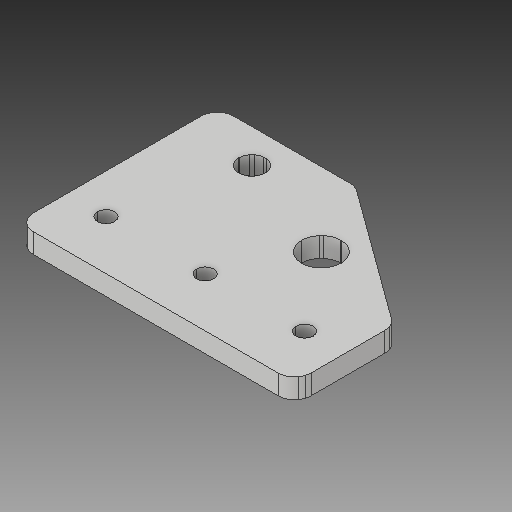
# Autodesk Inventor part: RearZHolder
Saved by Autodesk Inventor 2018 (Build 220112000, 112)
## iProperties
Created: 2016-07-23
Part Number: RearZHolder
Material: Generic
Document SubType Name: Modeling
Designer: joshm_000
Density: 1 g/cm^3
Appearance: Default
Author: joshm_000
Autodesk Inventor part; units mm, degrees
ref_plane "YZ Plane" through (0, 0, 0) normal (1, 0, 0) x (0, 1, 0)
ref_plane "XZ Plane" through (0, 0, 0) normal (0, 1, 0) x (-1, 0, 0)
ref_plane "XY Plane" through (0, 0, 0) normal (0, 0, 1) x (1, 0, 0)
sketch "Sketch1" plane through (0, 0, 0) normal (0, 1, 0) x (-1, 0, 0)
  line L0 (84.9035, 235.5734) -> (84.9035, 213.1177)
  spline S0 degree 3 poles (84.9035, 213.1177) (84.9035, 212.592) (84.9859, 212.0727) (85.1485, 211.5726) knots 1 1 1 1 2 2 2 2
  line L1 (84.9035, 213.1177) -> (84.9035, 212.592) construction
  line L2 (84.9035, 212.592) -> (84.9859, 212.0727) construction
  line L3 (84.9859, 212.0727) -> (85.1485, 211.5726) construction
  spline S1 degree 3 poles (85.1485, 211.5726) (85.3107, 211.0726) (85.5495, 210.6042) (85.8585, 210.1787) knots 2 2 2 2 3 3 3 3
  line L4 (85.1485, 211.5726) -> (85.3107, 211.0726) construction
  line L5 (85.3107, 211.0726) -> (85.5495, 210.6042) construction
  line L6 (85.5495, 210.6042) -> (85.8585, 210.1787) construction
  spline S2 degree 3 poles (85.8585, 210.1787) (86.1665, 209.755) (86.5368, 209.3843) (86.9604, 209.0756) knots 3 3 3 3 4 4 4 4
  line L7 (85.8585, 210.1787) -> (86.1665, 209.755) construction
  line L8 (86.1665, 209.755) -> (86.5368, 209.3843) construction
  line L9 (86.5368, 209.3843) -> (86.9604, 209.0756) construction
  line L10 (86.9604, 209.0756) -> (125.9367, 180.6949)
  spline S3 degree 3 poles (125.9367, 180.6949) (126.3618, 180.3855) (126.83, 180.1463) (127.3299, 179.9832) knots 5 5 5 5 6 6 6 6
  line L11 (125.9367, 180.6949) -> (126.3618, 180.3855) construction
  line L12 (126.3618, 180.3855) -> (126.83, 180.1463) construction
  line L13 (126.83, 180.1463) -> (127.3299, 179.9832) construction
  spline S4 degree 3 poles (127.3299, 179.9832) (127.8315, 179.8197) (128.3524, 179.7368) (128.88, 179.7368) knots 6 6 6 6 7 7 7 7
  line L14 (127.3299, 179.9832) -> (127.8315, 179.8197) construction
  line L15 (127.8315, 179.8197) -> (128.3524, 179.7368) construction
  line L16 (128.3524, 179.7368) -> (128.88, 179.7368) construction
  line L17 (128.88, 179.7368) -> (159.2657, 179.7368)
  line L18 (159.2657, 179.7368) -> (164.1855, 179.7368)
  spline S5 degree 3 poles (164.1855, 179.7368) (164.7112, 179.7368) (165.2304, 179.8192) (165.7305, 179.9816) (166.2305, 180.144) (166.6989, 180.3828) (167.1243, 180.6918) knots 9 9 9 9 10 10 10 11 11 11 11
  line L19 (164.1855, 179.7368) -> (164.7112, 179.7368) construction
  line L20 (164.7112, 179.7368) -> (165.2304, 179.8192) construction
  line L21 (165.2304, 179.8192) -> (165.7305, 179.9816) construction
  line L22 (165.7305, 179.9816) -> (166.2305, 180.144) construction
  line L23 (166.2305, 180.144) -> (166.6989, 180.3828) construction
  line L24 (166.6989, 180.3828) -> (167.1243, 180.6918) construction
  spline S6 degree 3 poles (167.1243, 180.6918) (167.5496, 181.0008) (167.9215, 181.3726) (168.2306, 181.798) knots 11 11 11 11 12 12 12 12
  line L25 (167.1243, 180.6918) -> (167.5496, 181.0008) construction
  line L26 (167.5496, 181.0008) -> (167.9215, 181.3726) construction
  line L27 (167.9215, 181.3726) -> (168.2306, 181.798) construction
  spline S7 degree 3 poles (168.2306, 181.798) (168.5396, 182.2232) (168.7783, 182.6917) (168.9408, 183.1919) knots 12 12 12 12 13 13 13 13
  line L28 (168.2306, 181.798) -> (168.5396, 182.2232) construction
  line L29 (168.5396, 182.2232) -> (168.7783, 182.6917) construction
  line L30 (168.7783, 182.6917) -> (168.9408, 183.1919) construction
  spline S8 degree 3 poles (168.9408, 183.1919) (169.103, 183.6918) (169.1854, 184.211) (169.1854, 184.7369) knots 13 13 13 13 14 14 14 14
  line L31 (168.9408, 183.1919) -> (169.103, 183.6918) construction
  line L32 (169.103, 183.6918) -> (169.1854, 184.211) construction
  line L33 (169.1854, 184.211) -> (169.1854, 184.7369) construction
  line L34 (169.1854, 184.7369) -> (169.1854, 235.5734)
  spline S9 degree 3 poles (169.1854, 235.5734) (169.1854, 236.0991) (169.103, 236.6185) (168.9408, 237.1183) knots 15 15 15 15 16 16 16 16
  line L35 (169.1854, 235.5734) -> (169.1854, 236.0991) construction
  line L36 (169.1854, 236.0991) -> (169.103, 236.6185) construction
  line L37 (169.103, 236.6185) -> (168.9408, 237.1183) construction
  spline S10 degree 3 poles (168.9408, 237.1183) (168.7783, 237.6186) (168.5396, 238.0869) (168.2306, 238.5122) knots 16 16 16 16 17 17 17 17
  line L38 (168.9408, 237.1183) -> (168.7783, 237.6186) construction
  line L39 (168.7783, 237.6186) -> (168.5396, 238.0869) construction
  line L40 (168.5396, 238.0869) -> (168.2306, 238.5122) construction
  spline S11 degree 3 poles (168.2306, 238.5122) (167.9215, 238.9377) (167.5496, 239.3094) (167.1243, 239.6184) knots 17 17 17 17 18 18 18 18
  line L41 (168.2306, 238.5122) -> (167.9215, 238.9377) construction
  line L42 (167.9215, 238.9377) -> (167.5496, 239.3094) construction
  line L43 (167.5496, 239.3094) -> (167.1243, 239.6184) construction
  spline S12 degree 3 poles (167.1243, 239.6184) (166.6989, 239.9275) (166.2305, 240.1662) (165.7305, 240.3287) (165.2304, 240.4911) (164.7112, 240.5734) (164.1855, 240.5734) knots 18 18 18 18 19 19 19 20 20 20 20
  line L44 (167.1243, 239.6184) -> (166.6989, 239.9275) construction
  line L45 (166.6989, 239.9275) -> (166.2305, 240.1662) construction
  line L46 (166.2305, 240.1662) -> (165.7305, 240.3287) construction
  line L47 (165.7305, 240.3287) -> (165.2304, 240.4911) construction
  line L48 (165.2304, 240.4911) -> (164.7112, 240.5734) construction
  line L49 (164.7112, 240.5734) -> (164.1855, 240.5734) construction
  line L50 (164.1855, 240.5734) -> (160.1854, 240.5734)
  line L51 (160.1854, 240.5734) -> (121.7853, 240.5734)
  line L52 (121.7853, 240.5734) -> (116.8657, 240.5734)
  line L53 (116.8657, 240.5734) -> (89.9037, 240.5734)
  spline S13 degree 3 poles (89.9037, 240.5734) (89.378, 240.5734) (88.8587, 240.4911) (88.3586, 240.3287) (87.8585, 240.1662) (87.3902, 239.9275) (86.9647, 239.6184) (86.5392, 239.3094) (86.1675, 238.9377) (85.8585, 238.5122) knots 24 24 24 24 25 25 25 26 26 26 27 27 27 27
  line L54 (89.9037, 240.5734) -> (89.378, 240.5734) construction
  line L55 (89.378, 240.5734) -> (88.8587, 240.4911) construction
  line L56 (88.8587, 240.4911) -> (88.3586, 240.3287) construction
  line L57 (88.3586, 240.3287) -> (87.8585, 240.1662) construction
  line L58 (87.8585, 240.1662) -> (87.3902, 239.9275) construction
  line L59 (87.3902, 239.9275) -> (86.9647, 239.6184) construction
  line L60 (86.9647, 239.6184) -> (86.5392, 239.3094) construction
  line L61 (86.5392, 239.3094) -> (86.1675, 238.9377) construction
  line L62 (86.1675, 238.9377) -> (85.8585, 238.5122) construction
  spline S14 degree 3 poles (85.8585, 238.5122) (85.5495, 238.0869) (85.3107, 237.6186) (85.1485, 237.1183) knots 27 27 27 27 28 28 28 28
  line L63 (85.8585, 238.5122) -> (85.5495, 238.0869) construction
  line L64 (85.5495, 238.0869) -> (85.3107, 237.6186) construction
  line L65 (85.3107, 237.6186) -> (85.1485, 237.1183) construction
  spline S15 degree 3 poles (85.1485, 237.1183) (84.9859, 236.6185) (84.9035, 236.0991) (84.9035, 235.5734) knots 28 28 28 28 29 29 29 29
  line L66 (85.1485, 237.1183) -> (84.9859, 236.6185) construction
  line L67 (84.9859, 236.6185) -> (84.9035, 236.0991) construction
  line L68 (84.9035, 236.0991) -> (84.9035, 235.5734) construction
  spline S16 degree 3 poles (148.4965, 185.9511) (146.2875, 185.9511) (144.4966, 187.7419) (144.4966, 189.9512) (144.4966, 192.1602) (146.2875, 193.951) (148.4965, 193.951) (150.7057, 193.951) (152.4966, 192.1602) (152.4966, 189.9512) (152.4966, 187.7419) (150.7057, 185.9511) (148.4965, 185.9511) knots 0 0 0 0 1 1 1 2 2 2 3 3 3 4 4 4 4
  line L69 (148.4965, 185.9511) -> (146.2875, 185.9511) construction
  line L70 (146.2875, 185.9511) -> (144.4966, 187.7419) construction
  line L71 (144.4966, 187.7419) -> (144.4966, 189.9512) construction
  line L72 (144.4966, 189.9512) -> (144.4966, 192.1602) construction
  line L73 (144.4966, 192.1602) -> (146.2875, 193.951) construction
  line L74 (146.2875, 193.951) -> (148.4965, 193.951) construction
  line L75 (148.4965, 193.951) -> (150.7057, 193.951) construction
  line L76 (150.7057, 193.951) -> (152.4966, 192.1602) construction
  line L77 (152.4966, 192.1602) -> (152.4966, 189.9512) construction
  line L78 (152.4966, 189.9512) -> (152.4966, 187.7419) construction
  line L79 (152.4966, 187.7419) -> (150.7057, 185.9511) construction
  line L80 (150.7057, 185.9511) -> (148.4965, 185.9511) construction
  spline S17 degree 3 poles (96.9036, 222.9735) (95.4677, 222.9735) (94.3038, 224.1376) (94.3038, 225.5735) (94.3038, 227.0094) (95.4677, 228.1735) (96.9036, 228.1735) (98.3397, 228.1735) (99.5037, 227.0094) (99.5037, 225.5735) (99.5037, 224.1376) (98.3397, 222.9735) (96.9036, 222.9735) knots 0 0 0 0 1 1 1 2 2 2 3 3 3 4 4 4 4
  line L81 (96.9036, 222.9735) -> (95.4677, 222.9735) construction
  line L82 (95.4677, 222.9735) -> (94.3038, 224.1376) construction
  line L83 (94.3038, 224.1376) -> (94.3038, 225.5735) construction
  line L84 (94.3038, 225.5735) -> (94.3038, 227.0094) construction
  line L85 (94.3038, 227.0094) -> (95.4677, 228.1735) construction
  line L86 (95.4677, 228.1735) -> (96.9036, 228.1735) construction
  line L87 (96.9036, 228.1735) -> (98.3397, 228.1735) construction
  line L88 (98.3397, 228.1735) -> (99.5037, 227.0094) construction
  line L89 (99.5037, 227.0094) -> (99.5037, 225.5735) construction
  line L90 (99.5037, 225.5735) -> (99.5037, 224.1376) construction
  line L91 (99.5037, 224.1376) -> (98.3397, 222.9735) construction
  line L92 (98.3397, 222.9735) -> (96.9036, 222.9735) construction
  spline S18 degree 3 poles (157.1854, 222.9735) (155.7495, 222.9735) (154.5854, 224.1376) (154.5854, 225.5735) (154.5854, 227.0094) (155.7495, 228.1735) (157.1854, 228.1735) (158.6213, 228.1735) (159.7854, 227.0094) (159.7854, 225.5735) (159.7854, 224.1376) (158.6213, 222.9735) (157.1854, 222.9735) knots 0 0 0 0 1 1 1 2 2 2 3 3 3 4 4 4 4
  line L93 (157.1854, 222.9735) -> (155.7495, 222.9735) construction
  line L94 (155.7495, 222.9735) -> (154.5854, 224.1376) construction
  line L95 (154.5854, 224.1376) -> (154.5854, 225.5735) construction
  line L96 (154.5854, 225.5735) -> (154.5854, 227.0094) construction
  line L97 (154.5854, 227.0094) -> (155.7495, 228.1735) construction
  line L98 (155.7495, 228.1735) -> (157.1854, 228.1735) construction
  line L99 (157.1854, 228.1735) -> (158.6213, 228.1735) construction
  line L100 (158.6213, 228.1735) -> (159.7854, 227.0094) construction
  line L101 (159.7854, 227.0094) -> (159.7854, 225.5735) construction
  line L102 (159.7854, 225.5735) -> (159.7854, 224.1376) construction
  line L103 (159.7854, 224.1376) -> (158.6213, 222.9735) construction
  line L104 (158.6213, 222.9735) -> (157.1854, 222.9735) construction
  spline S19 degree 3 poles (127.0446, 222.9735) (125.6087, 222.9735) (124.4446, 224.1376) (124.4446, 225.5735) (124.4446, 227.0094) (125.6087, 228.1735) (127.0446, 228.1735) (128.4805, 228.1735) (129.6446, 227.0094) (129.6446, 225.5735) (129.6446, 224.1376) (128.4805, 222.9735) (127.0446, 222.9735) knots 0 0 0 0 1 1 1 2 2 2 3 3 3 4 4 4 4
  line L105 (127.0446, 222.9735) -> (125.6087, 222.9735) construction
  line L106 (125.6087, 222.9735) -> (124.4446, 224.1376) construction
  line L107 (124.4446, 224.1376) -> (124.4446, 225.5735) construction
  line L108 (124.4446, 225.5735) -> (124.4446, 227.0094) construction
  line L109 (124.4446, 227.0094) -> (125.6087, 228.1735) construction
  line L110 (125.6087, 228.1735) -> (127.0446, 228.1735) construction
  line L111 (127.0446, 228.1735) -> (128.4805, 228.1735) construction
  line L112 (128.4805, 228.1735) -> (129.6446, 227.0094) construction
  line L113 (129.6446, 227.0094) -> (129.6446, 225.5735) construction
  line L114 (129.6446, 225.5735) -> (129.6446, 224.1376) construction
  line L115 (129.6446, 224.1376) -> (128.4805, 222.9735) construction
  line L116 (128.4805, 222.9735) -> (127.0446, 222.9735) construction
  spline S20 degree 3 poles (148.4965, 186.201) (146.4255, 186.201) (144.7465, 187.88) (144.7465, 189.9512) (144.7465, 192.022) (146.4255, 193.701) (148.4965, 193.701) (150.5677, 193.701) (152.2465, 192.022) (152.2465, 189.9512) (152.2465, 187.88) (150.5677, 186.201) (148.4965, 186.201) knots 0 0 0 0 1 1 1 2 2 2 3 3 3 4 4 4 4
  line L117 (148.4965, 186.201) -> (146.4255, 186.201) construction
  line L118 (146.4255, 186.201) -> (144.7465, 187.88) construction
  line L119 (144.7465, 187.88) -> (144.7465, 189.9512) construction
  line L120 (144.7465, 189.9512) -> (144.7465, 192.022) construction
  line L121 (144.7465, 192.022) -> (146.4255, 193.701) construction
  line L122 (146.4255, 193.701) -> (148.4965, 193.701) construction
  line L123 (148.4965, 193.701) -> (150.5677, 193.701) construction
  line L124 (150.5677, 193.701) -> (152.2465, 192.022) construction
  line L125 (152.2465, 192.022) -> (152.2465, 189.9512) construction
  line L126 (152.2465, 189.9512) -> (152.2465, 187.88) construction
  line L127 (152.2465, 187.88) -> (150.5677, 186.201) construction
  line L128 (150.5677, 186.201) -> (148.4965, 186.201) construction
  spline S21 degree 3 poles (115.2365, 196.1224) (111.9229, 196.1224) (109.2366, 198.8089) (109.2366, 202.1224) (109.2366, 205.4362) (111.9229, 208.1224) (115.2365, 208.1224) (118.5502, 208.1224) (121.2365, 205.4362) (121.2365, 202.1224) (121.2365, 198.8089) (118.5502, 196.1224) (115.2365, 196.1224) knots 0 0 0 0 1 1 1 2 2 2 3 3 3 4 4 4 4
  line L129 (115.2365, 196.1224) -> (111.9229, 196.1224) construction
  line L130 (111.9229, 196.1224) -> (109.2366, 198.8089) construction
  line L131 (109.2366, 198.8089) -> (109.2366, 202.1224) construction
  line L132 (109.2366, 202.1224) -> (109.2366, 205.4362) construction
  line L133 (109.2366, 205.4362) -> (111.9229, 208.1224) construction
  line L134 (111.9229, 208.1224) -> (115.2365, 208.1224) construction
  line L135 (115.2365, 208.1224) -> (118.5502, 208.1224) construction
  line L136 (118.5502, 208.1224) -> (121.2365, 205.4362) construction
  line L137 (121.2365, 205.4362) -> (121.2365, 202.1224) construction
  line L138 (121.2365, 202.1224) -> (121.2365, 198.8089) construction
  line L139 (121.2365, 198.8089) -> (118.5502, 196.1224) construction
  line L140 (118.5502, 196.1224) -> (115.2365, 196.1224) construction
  point P0 (0, 0)
  constraints: 18 end point, 60 other
extrude "Extrusion1" add sketch "Sketch1" along normal blind 6 contours S15 S14 S13 L53 L52 L51 L50 S12 S11 S10 S9 L34 S8 S7 S6 S5 L18 L17 S4 S3 L10 S2 S1 S0 L0
sketch "Sketch2" plane through (0, 6, 0) normal (0, 1, 0) x (1, 0, 0)
  line L0 (-86.9604, -209.0756) -> (-125.9367, -180.6949) projected
  line L1 (-128.88, -179.7368) -> (-164.1855, -179.7368) projected
  line L2 (-169.1854, -184.7369) -> (-169.1854, -235.5734) projected
  line L3 (-164.1855, -240.5734) -> (-89.9037, -240.5734) projected
  line L4 (-84.9035, -235.5734) -> (-84.9035, -213.1177) projected
  line L5 (-159.7853, -225.5529) -> (-154.5855, -225.5529)
  line L6 (-129.6445, -225.5529) -> (-124.4447, -225.5529)
  line L7 (-99.5036, -225.5529) -> (-94.3039, -225.5529)
  point P0 (0, 0)
  point P1 (-115.2365, -196.1224)
  point P2 (-148.4965, -185.9511)
  point P3 (-127.0446, -222.9735)
  point P4 (-157.1854, -222.9735)
  point P5 (-96.9036, -222.9735)
  point P6 (-85.1485, -211.5726)
  point P7 (-85.8585, -210.1787)
  point P8 (-127.3299, -179.9832)
  point P9 (-167.1243, -180.6918)
  point P10 (-168.2306, -181.798)
  point P11 (-168.9408, -183.1919)
  point P12 (-168.9408, -237.1183)
  point P13 (-168.2306, -238.5122)
  point P14 (-167.1243, -239.6184)
  point P15 (-85.8585, -238.5122)
  point P16 (-85.1485, -237.1183)
  point P17 (-157.1854, -225.5529)
  point P18 (-127.0446, -225.5529)
  point P19 (-96.9037, -225.5529)
  constraints: 6 end point, 4 point on line, 3 midpoint, 1 horizontal, 27 other
hole "Hole1" at (-157.1854, 6, 225.5529) at (-127.0446, 6, 225.5529) at (-96.9037, 6, 225.5529) direction (0, -1, 0) diameter 5.2 end through all
sketch "Sketch3" plane through (0, 6, 0) normal (0, 1, 0) x (1, 0, 0)
  line L0 (-115.2365, -208.1224) -> (-115.2365, -196.1224)
  line L1 (-148.4965, -193.951) -> (-148.4965, -185.9511)
  circle A0 centre (-148.4965, -189.951) radius 4.0002
  point P0 (0, 0)
  constraints: 4 end point, 2 vertical, 2 vertical alignment, 1 centre point, 1 midpoint, 2 other
extrude "Extrusion2" cut sketch "Sketch3" against normal blind 10
sketch "Sketch5" plane through (0, 6, 0) normal (0, 1, 0) x (1, 0, 0)
  circle A0 centre (-115.2365, -202.1224) radius 6
  point P0 (0, 0)
  point P1 (-115.2365, -196.1224)
  dimension "d11" = 12
  constraints: 1 centre point, 1 other
  measures "d11" diameter of A0
extrude "Extrusion3" cut sketch "Sketch5" against normal blind 10
body "Solid1"
